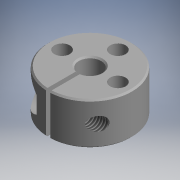
# Autodesk Inventor part: SCST8-15b
Saved by Autodesk Inventor 2017.3 (Build 213256000, 256)
## iProperties
Part Number: SCST8-15b
Material: Generic
Catalog Web Link: www.cadenas.de
Description: SCST, PSCST, SSCST, SCSTR, PSCSTR, SSCSTR-b-Shaft Collars - 3 Holes/3 Taps
Vendor: MISUMI
Document SubType Name: Modeling
Designer: partserver
Manufacturer: MISUMI
Mass: 7.4266 g
Surface Area: 42.3927 cm^2
Volume: 7.4266 cm^3
Density: 1 g/cm^3
Appearance: PSOLRGB-192-192-192
Category: PARTsolutions
Company: MISUMI
Title: SCST8-15
Author: Cadenas PARTsolutions
Comments: Shaft Collars - 3 Holes/3 Taps
PSOL_IDENT_0: {$CADENAS_DATA\23d-libs\misumi\metric\03_set_collars\scst\scst_b.prj},208 {VTYP=3D},{NB=SCST8-15b},{
PSOL_IDENT_1: LINA=SCST8-15},{NN=SCST, PSCST, SSCST, SCSTR, PSCSTR, SSCSTR-b},{DATE=30.06.2021 12:52:04},{GEOMDATE=
PSOL_IDENT_2: 30.10.2015 01:43:51},{VERSION=},{LINEID=50},{WBVAR=TS,MAT,ST,BS},{WBNUMERIC=BS}  {NB=SCST8-15b},{LIN
PSOL_IDENT_3: A=SCST8-15},{KT=DUMMY},{PN=SCST8-15},{TYPE=SCST},{TS=3H},{TSALG= '3H' , '3-Hole' , '3T' , '3-Tapped'
PSOL_IDENT_4: },{TSA='3H', '3-Hole'},{MAT=S45C},{ST=BO},{STALG= 'BO' , 'Black Oxide' , 'ENP' , 'Electroless Nicke
PSOL_IDENT_5: l Plating' },{AC=Hex Socket Head Cap Screw 1 pc.},{ACMAT=4137 Alloy Steel},{D=8},{BS=15},{BALG= 8 ,
PSOL_IDENT_6: 10 , 15 },{D1=30},{M=M6},{M3D=6},{DD=6.6},{R=6.00},{W=1.5},{X=9.0},{Y=5},{P=20},{C=0.5},{S=5.5},{M1=
PSOL_IDENT_7: -},{M13D=0},{L=15}
NB: SCST8-15b
NN: SCST, PSCST, SSCST, SCSTR, PSCSTR, SSCSTR-b
NT: Shaft Collars - 3 Holes/3 Taps
NBSYN: $PN.b
LINA: SCST8-15
CATALOG: Misumi
PN: SCST8-15
TS: 3-Hole
MAT: 1045 Carbon Steel
ST: Black Oxide
AC: Hex Socket Head Cap Screw 1 pc.
ACMAT: 4137 Alloy Steel
D: 8
BS: 15
D1: 30
M: M6
DD: 6.6
R: 6
W: 1.5
X: 9
Y: 5
P: 20
C: 0.5
S: 5.5
M1: -
SUPPLIER: MISUMI
ARTICLENO: SCST8-15b
BOMINFO: SCST8-15
CREATOR: CADENAS GmbH
Autodesk Inventor part; units mm, degrees
sketch "Sketch_14" plane through (0, 0, 0) normal (1, 0, 0) x (0, 1, 0)
  line L0 (0, -7.5) -> (0, 7.5)
  line L1 (0, 7.5) -> (14.5, 7.5)
  line L2 (14.5, 7.5) -> (15, 7)
  line L3 (15, 7) -> (15, -7)
  line L4 (15, -7) -> (14.5, -7.5)
  line L5 (14.5, -7.5) -> (0, -7.5)
  line L6 (0, -7.5) -> (0, 7.5)
  constraints: 14 end point
revolve "Revolution1" add sketch "Sketch_14" angle 360 about axis through (0, 0, -7.5) along (0, 0, -1)
sketch "Sketch_15" plane through (0, 0, 0) normal (1, 0, 0) x (0, 1, 0)
  line L0 (0, -7.5) -> (0, 7.5)
  line L1 (0, 7.5) -> (4.5, 7.5)
  line L2 (4.5, 7.5) -> (4, 7)
  line L3 (4, 7) -> (4, -7)
  line L4 (4, -7) -> (4.5, -7.5)
  line L5 (4.5, -7.5) -> (0, -7.5)
  line L6 (0, -7.5) -> (0, 7.5)
  constraints: 14 end point
revolve "Revolution2" cut sketch "Sketch_15" angle 360 about axis through (0, 0, -7.5) along (0, 0, -1)
sketch "Sketch_16" plane through (0, 0, 0) normal (0, 0, 1) x (1, 0, 0)
  arc A0 (-0.75, -15.9824) -> (0.75, -15.9824) centre (0, 0) ccw
  line L0 (0.75, -15.9824) -> (0.75, 0)
  line L1 (0.75, 0) -> (-0.75, 0)
  line L2 (-0.75, 0) -> (-0.75, -15.9824)
  constraints: 6 end point, 2 point on circle, 1 centre point
extrude "Extrusion1" cut sketch "Sketch_16" along normal mid plane 15
sketch "Sketch4" plane through (0, 0, -7.5) normal (0, 0, -1) x (-1, 0, 0)
  point P0 (-10, 0)
hole "Hole1" at (10, 0, -7.5) direction (0, 0, 1) diameter 5.5 depth 15
sketch "Sketch5" plane through (0, 0, -7.5) normal (0, 0, -1) x (-1, 0, 0)
  point P0 (10, 0)
hole "Hole2" at (-10, 0, -7.5) direction (0, 0, 1) diameter 5.5 depth 15
sketch "Sketch6" plane through (0, 0, -7.5) normal (0, 0, -1) x (-1, 0, 0)
  point P0 (0, 10)
hole "Hole3" at (0, 10, -7.5) direction (0, 0, 1) diameter 5.5 depth 15
sketch "Sketch_23" plane through (0, -9, 0) normal (0, 1, 0) x (1, 0, 0)
  line L0 (15, 0) -> (0, 0)
  line L1 (0, 0) -> (0, 3.3)
  line L2 (0, 3.3) -> (5, 3.3)
  line L3 (5, 3.3) -> (5, 6)
  line L4 (5, 6) -> (15, 6)
  line L5 (15, 6) -> (15, 0)
  line L6 (15, 0) -> (0, 0)
  constraints: 14 end point
revolve "Revolution3" cut sketch "Sketch_23" angle 360 about axis through (15, -9, 0) along (1, 0, 0)
sketch "Sketch_25" plane through (0, 0, 0) normal (0, 0, 1) x (1, 0, 0)
  line L0 (-0.75, -9) -> (-13.7477, -9)
  line L1 (-13.7477, -9) -> (-13.7477, -6.5415)
  line L2 (-13.7477, -6.5415) -> (-1.2915, -6.5415)
  line L3 (-1.2915, -6.5415) -> (-0.75, -6)
  line L4 (-0.75, -6) -> (-0.75, -9)
  line L5 (-0.75, -9) -> (-13.7477, -9)
  constraints: 12 end point
revolve "Revolution4" cut sketch "Sketch_25" angle 360 about axis through (-0.75, -9, 0) along (1, 0, 0)
thread "Thread1" size "M6x1" class "6H" standard "ISO Metric profile" length 12.4562
ref_plane "to_bolt_XY" through (5, -9, 0) normal (1, 0, 0) x (0, 0, -1)
ref_plane "to_bolt_YZ" through (5, -9, 0) normal (0, 0, -1) x (0, 1, 0)
ref_plane "to_bolt_ZX" through (5, -9, 0) normal (0, 1, 0) x (1, 0, 0)
body "Solid1"
